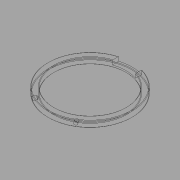
# Autodesk Inventor part: KE-SP-02-P1
Saved by Autodesk Inventor 2018 (Build 220112000, 112)
## iProperties
Created: 2015-08-04
Part Number: KE-SP-02-P1
Material: 一般
Document SubType Name: Modeling
Designer: ERIC
Density: 1 g/cm^3
Appearance: 預設
Author: ERIC
Autodesk Inventor part; units mm, degrees
sketch "草圖1" plane through (0, 0, 0) normal (0, 0, 1) x (1, 0, 0)
  circle A0 centre (0, 0) radius 39.9
  circle A1 centre (0, 0) radius 34.1
  dimension "d0" = 79.8
  dimension "d3" = 68.2
  constraints: 2 centre point, 2 coincident
  measures "d0" diameter of A0
  measures "d3" diameter of A1
extrude "擠出1" add sketch "草圖1" along normal blind 6
sketch "草圖2" plane through (0, 0, 6) normal (0, 0, 1) x (1, 0, 0)
  circle A0 centre (0, 0) radius 34.1 projected
  circle A1 centre (0, 0) radius 39.9 projected
  line L0 (0, 0) -> (0, 39.9)
  line L1 (11, 40.6521) -> (11, 12.8237)
  line L2 (-11, 40.6521) -> (-11, 12.8237)
  line L3 (-11, 40.6521) -> (11, 40.6521)
  line L4 (-11, 12.8237) -> (11, 12.8237)
  point P0 (11, 38.3537)
  point P1 (11, 32.2771)
  point P2 (-11, 38.3537)
  point P3 (-11, 32.2771)
  dimension "d6" = 22
  constraints: 10 end point, 5 point on circle, 4 point on line, 2 horizontal, 2 parallel, 1 vertical, 1 other
  measures "d6" distance between parallel lines of L1 L2
extrude "擠出2" cut sketch "草圖2" against normal blind 4 contours A0 L0 A1 L1 | L2 A1 L0 A0
ref_plane "工作平面1" through (0, 0, 3) normal (0, 0, 1) x (1, 0, 0)
sketch "草圖3" plane through (0, 0, 3) normal (0, 0, 1) x (1, 0, 0)
  line L0 (0, 0) -> (0, -42.4806)
  line L1 (0, 0) -> (-20.55, -34.201)
  line L2 (0, 0) -> (20.55, -34.201)
  arc A0 (-11, 38.3537) -> (11, 38.3537) centre (0, 0) ccw projected
  line L3 (-20.55, -34.201) -> (20.55, -34.201)
  dimension "d27" = 31
  constraints: 8 end point, 2 point on circle, 1 perpendicular, 1 vertical, 1 other
  measures "d27" angle of L1 L0
ref_plane "工作平面2" through (20.55, -34.201, 3) normal (0.515, -0.8572, 0) x (0.8572, 0.515, 0)
ref_plane "工作平面3" through (-20.55, -34.201, 3) normal (-0.515, -0.8572, 0) x (0.8572, -0.515, 0)
sketch "草圖4" plane through (20.55, -34.201, 3) normal (0.515, -0.8572, 0) x (0.8572, 0.515, 0)
  point P0 (0, -3)
  point P1 (0, 0)
hole "孔1" at (20.55, -34.201, 3) direction (-0.515, 0.8572, 0) diameter 3 depth 3.5 tip angle 118
sketch "草圖5" plane through (-20.55, -34.201, 3) normal (-0.515, -0.8572, 0) x (0.8572, -0.515, 0)
  point P0 (0, -3)
  point P1 (0, 0)
hole "孔2" at (-20.55, -34.201, 3) direction (0.515, 0.8572, 0) diameter 3 depth 3.5 tip angle 118
chamfer "倒角1" distance 0.5 angle 45 6 edges at (-19.8458, -27.73, 6) (27.73, 19.8458, 6) (-34.1, 0, 0) (-24.0116, -31.8662, 6) (31.8662, 24.0116, 6) (-39.9, 0, 0)
